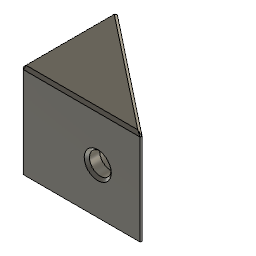
cable_chain_mount_gantry v0 (Autodesk Fusion 360 design; units mm, degrees)
Autodesk Fusion 360 part; units mm, degrees
sketch "Sketch1" plane through (0, 0, 0) normal (0, 0, 1) x (1, 0, 0)
  line L0 (0, 0) -> (19, 0)
  line L1 (0, 0) -> (0, 15)
  line L2 (0, 15) -> (19, 0)
  dimension "d1" = 19
  dimension "d2" = 15
  constraint coincident L0.start L1.start
  constraint horizontal L0
  constraint perpendicular L0 L1
  measures "d1" distance of L0.start L0.end
  measures "d2" distance of L0.start L1.end
extrude "Extrude1" add sketch "Sketch1" along normal blind 15
sketch "cable_holes" plane through (0, 0, 0) normal (0, -1, 0) x (1, 0, 0)
  line L0 (0, 0) -> (19, 0)
  line L1 (19, 0) -> (19, 15)
  line L2 (19, 15) -> (0, 15)
  line L3 (0, 15) -> (0, 0)
  circle A0 centre (4.2, 10.7) radius 1.7
  circle A1 centre (4.2, 4.3) radius 1.7
  circle A2 centre (12, 7.5) radius 1.7
  line L4 (19, 7.5) -> (0, 7.5) construction
  circle A3 centre (4.2, 10.7) radius 3
  circle A4 centre (4.2, 4.3) radius 3
  circle A5 centre (12, 7.5) radius 3
  dimension "d7" = 3.4
  dimension "d8" = 3.4
  dimension "d9" = 3.4
  dimension "d10" = 4.2
  dimension "d11" = 4.2
  dimension "d12" = 6.4
  dimension "d13" = 12
  dimension "d14" = 4.3
  dimension "d20" = 6
  dimension "d21" = 6
  dimension "d22" = 6
  constraint midpoint L1 L4.start
  constraint midpoint L3 L4.end
  constraint coincident A2.centre L4
  constraint concentric A0 A3
  constraint concentric A1 A4
  constraint concentric A2 A5
  measures "d7" diameter of A0
  measures "d8" diameter of A1
  measures "d9" diameter of A2
  measures "d10" distance of L3 A0.centre
  measures "d11" distance of L3 A1.centre
  measures "d12" distance of A0.centre A1.centre
  measures "d13" distance of L3 A2.centre
  measures "d14" distance of L2 A0.centre
  measures "d20" diameter of A3
  measures "d21" diameter of A4
  measures "d22" diameter of A5
extrude "Extrude2" cut sketch "cable_holes" against normal blind 15 contours A2 | A5
extrude "Extrude4" add sketch "cable_holes" against normal blind 2 contours A5
sketch "Sketch3" plane through (0, 0, 0) normal (-1, 0, 0) x (0, -1, 0)
  line L0 (-15, 0) -> (0, 0)
  line L1 (0, 0) -> (0, 15)
  line L2 (0, 15) -> (-15, 15)
  line L3 (-15, 15) -> (-15, 0)
  circle A0 centre (-7.5, 7.5) radius 1.7
  line L4 (-7.5, 15) -> (-7.5, 0) construction
  line L5 (-15, 7.5) -> (0, 7.5) construction
  circle A1 centre (-7.5, 7.5) radius 3
  dimension "d17" = 3.4
  dimension "d25" = 6
  constraint midpoint L2 L4.start
  constraint midpoint L0 L4.end
  constraint midpoint L3 L5.start
  constraint perpendicular L3 L5
  constraint midpoint A0.centre L4
  constraint concentric A0 A1
  measures "d17" diameter of A0
  measures "d25" diameter of A1
extrude "Extrude3" cut sketch "Sketch3" against normal blind 15 contours A0 | A1
extrude "Extrude5" add sketch "Sketch3" against normal blind 2 contours A1
chamfer "Chamfer1" distance 0.4 angle 45 4 edges at (15, 3.1579, 7.5) (5.7, 10.5, 7.5) (0, 9.085, 8.1147) (10.415, 0, 8.1147)
chamfer "Chamfer2" distance 0.4 angle 45 9 edges at (9.5, 7.5, 15) (0, 7.5, 15) (9.5, 0, 15) (19, 0, 7.5) (0, 15, 7.5) (0, 0, 7.5) (0, 7.5, 0) (9.5, 7.5, 0) (9.5, 0, 0)
equation "inner_hole = 3.4 mm"
equation "outer_hole = 6 mm"
equation "d7 = inner_hole"
equation "d8 = inner_hole"
equation "d9 = inner_hole"
equation "d13 = 4.2 mm + 7.8 mm"
equation "d17 = inner_hole"
equation "d20 = outer_hole"
equation "d21 = outer_hole"
equation "d22 = outer_hole"
equation "d25 = outer_hole"
